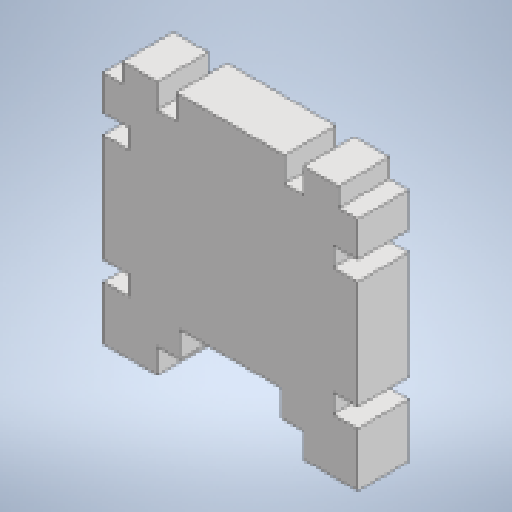
# Autodesk Inventor part: Contrapeso
Saved by Autodesk Inventor 2024 (Build 280153000, 153)
## iProperties
Created: 2024-07-16
Part Number: Contrapeso
Material: Genérico
Document SubType Name: Modeling
Designer: sergi
Density: 1 g/cm^3
Appearance: Valor por defecto
Author: sergi
Autodesk Inventor part; units mm, degrees
ref_plane "YZ Plane" through (0, 0, 0) normal (1, 0, 0) x (0, 1, 0)
ref_plane "XZ Plane" through (0, 0, 0) normal (0, 1, 0) x (-1, 0, 0)
ref_plane "XY Plane" through (0, 0, 0) normal (0, 0, 1) x (1, 0, 0)
sketch "Boceto1" plane through (0, 0, 0) normal (0, 0, 1) x (1, 0, 0)
  line L0 (0, -12.2) -> (0, -206) projected
  line L1 (-3, -206) -> (-3, -12.2) projected
  line L2 (0, -206) -> (-3, -206) projected
  line L3 (-206, -203) -> (-206, 0) projected
  line L4 (-203, 0) -> (-203, -203) projected
  line L5 (-206, 0) -> (-203, 0) projected
  line L6 (-203, -203) -> (-3, -203)
  line L7 (-3, -203) -> (-3, -3)
  line L8 (-3, -3) -> (-203, -3)
  line L9 (-203, -3) -> (-203, -203)
  line L10 (-103, -203) -> (-103, -163)
  line L11 (-103, -163) -> (-143, -163)
  line L12 (-143, -163) -> (-63, -163)
  line L13 (-63, -163) -> (-63, -203)
  line L14 (-63, -203) -> (-143, -203)
  line L15 (-143, -203) -> (-143, -163)
  line L16 (-147.5, -3) -> (-147.5, -20.5)
  line L17 (-158.5, -20.5) -> (-158.5, -3)
  line L18 (-147.5, -3) -> (-147.5, -20.5)
  line L19 (-158.5, -3) -> (-147.5, -3) projected
  circle A0 centre (-191, -53) radius 2.1 projected
  line L20 (-185.5, -58.5) -> (-203, -58.5) projected
  line L21 (-185.5, -47.5) -> (-185.5, -58.5) projected
  line L22 (-203, -47.5) -> (-185.5, -47.5) projected
  line L23 (-203, -58.5) -> (-203, -47.5) projected
  circle A1 centre (-53, -15) radius 2.1 projected
  line L24 (-58.5, -20.5) -> (-58.5, -3) projected
  line L25 (-47.5, -20.5) -> (-58.5, -20.5) projected
  line L26 (-47.5, -3) -> (-47.5, -20.5) projected
  line L27 (-58.5, -3) -> (-47.5, -3) projected
  circle A2 centre (-15, -53) radius 2.1 projected
  line L28 (-20.5, -47.5) -> (-3, -47.5) projected
  line L29 (-20.5, -58.5) -> (-20.5, -47.5) projected
  line L30 (-3, -58.5) -> (-20.5, -58.5) projected
  line L31 (-3, -47.5) -> (-3, -58.5) projected
  line L32 (-20.5, -147.5) -> (-3, -147.5) projected
  line L33 (-3, -158.5) -> (-20.5, -158.5) projected
  line L34 (-20.5, -158.5) -> (-20.5, -147.5) projected
  line L35 (-47.5, -185.5) -> (-47.5, -203) projected
  line L36 (-58.5, -203) -> (-58.5, -185.5) projected
  line L37 (-58.5, -185.5) -> (-47.5, -185.5) projected
  line L38 (-158.5, -203) -> (-158.5, -185.5) projected
  line L39 (-158.5, -185.5) -> (-147.5, -185.5) projected
  line L40 (-147.5, -185.5) -> (-147.5, -203) projected
  line L41 (-185.5, -158.5) -> (-203, -158.5) projected
  line L42 (-203, -147.5) -> (-185.5, -147.5) projected
  line L43 (-185.5, -147.5) -> (-185.5, -158.5) projected
  line L44 (-158.5, -3) -> (-147.5, -3)
  line L45 (-147.5, -3) -> (-147.5, -20.5)
  line L46 (-158.5, -20.5) -> (-158.5, -3)
  line L47 (-158.5, -3) -> (-147.5, -3)
  line L48 (-147.5, -3) -> (-147.5, -20.5)
  line L49 (-147.5, -20.5) -> (-158.5, -20.5)
  line L50 (-158.5, -20.5) -> (-158.5, -3)
  line L51 (-147.5, -22.5) -> (-160.5, -22.5)
  line L52 (-160.5, -22.5) -> (-160.5, -3)
  line L53 (-160.5, -3) -> (-145.5, -3)
  line L54 (-145.5, -3) -> (-145.5, -22.5)
  line L55 (-145.5, -22.5) -> (-160.5, -22.5)
  line L56 (-160.5, -22.5) -> (-160.5, -3)
  circle A3 centre (-103, -103) radius 47 projected
  line L57 (-47.5, -22.5) -> (-60.5, -22.5)
  line L58 (-60.5, -22.5) -> (-60.5, -3)
  line L59 (-45.5, -3) -> (-45.5, -22.5)
  line L60 (-45.5, -22.5) -> (-60.5, -22.5)
  line L61 (-60.5, -22.5) -> (-60.5, -3)
  line L62 (-183.5, -160.5) -> (-203, -160.5)
  line L63 (-203, -147.5) -> (-185.5, -147.5)
  line L64 (-203, -147.5) -> (-185.5, -147.5)
  line L65 (-185.5, -158.5) -> (-203, -158.5)
  line L66 (-183.5, -160.5) -> (-203, -160.5)
  line L67 (-185.5, -158.5) -> (-203, -158.5)
  line L68 (-185.5, -158.5) -> (-203, -158.5)
  line L69 (-183.5, -147.5) -> (-183.5, -160.5)
  line L70 (-203, -147.5) -> (-185.5, -147.5)
  line L71 (-203, -147.5) -> (-185.5, -147.5)
  line L72 (-185.5, -147.5) -> (-185.5, -158.5)
  line L73 (-183.5, -145.5) -> (-183.5, -160.5)
  line L74 (-203, -145.5) -> (-183.5, -145.5)
  line L75 (-183.5, -47.5) -> (-183.5, -60.5)
  line L76 (-183.5, -45.5) -> (-183.5, -60.5)
  line L77 (-183.5, -60.5) -> (-203, -60.5)
  line L78 (-183.5, -60.5) -> (-203, -60.5)
  line L79 (-203, -45.5) -> (-183.5, -45.5)
  line L80 (-45.5, -183.5) -> (-45.5, -203)
  line L81 (-58.5, -203) -> (-58.5, -185.5)
  line L82 (-58.5, -203) -> (-58.5, -185.5)
  line L83 (-47.5, -185.5) -> (-47.5, -203)
  line L84 (-45.5, -183.5) -> (-45.5, -203)
  line L85 (-47.5, -185.5) -> (-47.5, -203)
  line L86 (-47.5, -185.5) -> (-47.5, -203)
  line L87 (-58.5, -183.5) -> (-45.5, -183.5)
  line L88 (-58.5, -203) -> (-58.5, -185.5)
  line L89 (-58.5, -203) -> (-58.5, -185.5)
  line L90 (-58.5, -185.5) -> (-47.5, -185.5)
  line L91 (-60.5, -183.5) -> (-45.5, -183.5)
  line L92 (-60.5, -203) -> (-60.5, -183.5)
  line L93 (-158.5, -183.5) -> (-145.5, -183.5)
  line L94 (-160.5, -183.5) -> (-145.5, -183.5)
  line L95 (-145.5, -183.5) -> (-145.5, -203)
  line L96 (-145.5, -183.5) -> (-145.5, -203)
  line L97 (-160.5, -203) -> (-160.5, -183.5)
  line L98 (-22.5, -45.5) -> (-3, -45.5)
  line L99 (-3, -58.5) -> (-20.5, -58.5)
  line L100 (-3, -58.5) -> (-20.5, -58.5)
  line L101 (-20.5, -47.5) -> (-3, -47.5)
  line L102 (-22.5, -45.5) -> (-3, -45.5)
  line L103 (-20.5, -47.5) -> (-3, -47.5)
  line L104 (-20.5, -47.5) -> (-3, -47.5)
  line L105 (-22.5, -58.5) -> (-22.5, -45.5)
  line L106 (-3, -58.5) -> (-20.5, -58.5)
  line L107 (-3, -58.5) -> (-20.5, -58.5)
  line L108 (-20.5, -58.5) -> (-20.5, -47.5)
  line L109 (-22.5, -60.5) -> (-22.5, -45.5)
  line L110 (-3, -60.5) -> (-22.5, -60.5)
  line L111 (-22.5, -158.5) -> (-22.5, -145.5)
  line L112 (-22.5, -160.5) -> (-22.5, -145.5)
  line L113 (-22.5, -145.5) -> (-3, -145.5)
  line L114 (-22.5, -145.5) -> (-3, -145.5)
  line L115 (-3, -160.5) -> (-22.5, -160.5)
  line L116 (-145.5, -183.5) -> (-60.5, -183.5)
  line L117 (-3, -3) -> (-18, -3)
  line L118 (-18, -3) -> (-18, -18)
  line L119 (-18, -18) -> (-3, -18)
  line L120 (-3, -18) -> (-3, -3)
  line L121 (-203, -3) -> (-188, -3)
  line L122 (-188, -3) -> (-188, -18)
  line L123 (-188, -18) -> (-203, -18)
  line L124 (-203, -18) -> (-203, -3)
  line L125 (-206, -203) -> (-203, -203) projected
  line L126 (0, -12.2) -> (-3, -12.2) projected
  point P0 (0, 0)
  point P1 (-3, -203)
  point P2 (-3, -160.5)
  point P3 (-3, -145.5)
  point P4 (-3, -60.5)
  point P5 (-3, -45.5)
  point P6 (-63, -183.5)
  point P7 (-143, -183.5)
  point P8 (-3, -18)
  dimension "d3" = 40
  dimension "d4" = 40
  dimension "d5" = 80
  dimension "d6" = 2
  dimension "d7" = 15
  dimension "d8" = 15
  dimension "d11" = 360
  dimension "d13" = 15
  dimension "d14" = 15
  dimension "d15" = 15
  constraints: 188 end point, 14 parallel, 9 perpendicular, 7 horizontal, 1 midpoint, 1 point on line, 1 vertical, 154 other
  measures "d3" distance of L10.start L10.end
  measures "d4" distance of L10.end L11.end
  measures "d5" distance of L13.end L14.end
  measures "d6" distance between parallel lines of L49 L51
  measures "d7" distance of L54.end L55.end
  measures "d8" distance of L59.end L60.end
  measures "d13" distance of L118.end L117.end
  measures "d14" distance of L122.end L123.end
  measures "d15" distance of L121.end L122.end
extrude "Extrusión1" add sketch "Boceto1" against normal blind 40 contours L1 L98 L105 L109 L110 L113 L111 L112 L115 L6 L80 L87 L91 L116 L13 L12 L11 L15 L93 L94 L97 L4 L62 L69 L73 L74 L77 L75 L76 L79 L123 L122 L8 L52 L51 L55 L54 L58 L57 L60 L59 L118 L119 | A3
shell "Vaciado1" thickness 0.8 removed faces 1 at (-103, -69.3333, -40)
